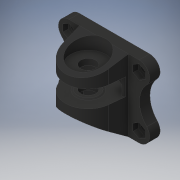
# Autodesk Inventor part: Y Bearing Mount
Saved by Autodesk Inventor 2020.2 (Build 242310000, 310)
## iProperties
Created: 2018-06-15
Part Number: Y Bearing Mount
Material: ABS Plastic
Document SubType Name: Modeling
Designer: Richard
Density: 1.06 g/cm^3
Appearance: Rubber - Black
Author: Richard
Autodesk Inventor part; units mm, degrees
ref_plane "YZ Plane" through (0, 0, 0) normal (1, 0, 0) x (0, 1, 0)
ref_plane "XZ Plane" through (0, 0, 0) normal (0, 1, 0) x (-1, 0, 0)
ref_plane "XY Plane" through (0, 0, 0) normal (0, 0, 1) x (1, 0, 0)
sketch "Sketch1" plane through (0, 0, 0) normal (0, 0, 1) x (1, 0, 0)
  line L0 (-20, -20.5) -> (20, -20.5)
  line L1 (20, -20.5) -> (20, 20.5) construction
  line L2 (20, 20.5) -> (-20, 20.5)
  line L3 (-20, 20.5) -> (-20, -20.5) construction
  line L4 (-20, -20.5) -> (20, 20.5) construction
  line L5 (20, -20.5) -> (-20, 20.5) construction
  arc A0 (-20, 20.5) -> (-24.3401, 10.3571) centre (-20, 14.5) ccw
  arc A1 (-24.3401, -10.3571) -> (-20, -20.5) centre (-20, -14.5) ccw
  arc A2 (20, -20.5) -> (24.3401, -10.3571) centre (20, -14.5) ccw
  arc A3 (24.3401, 10.3571) -> (20, 20.5) centre (20, 14.5) ccw
  arc A4 (-24.3401, -10.3571) -> (-24.3401, 10.3571) centre (-35.19, 0) ccw
  arc A5 (24.3401, 10.3571) -> (24.3401, -10.3571) centre (35.19, 0) ccw
  point P0 (0, 0)
  point P1 (-20, 14.5)
  point P2 (-20, -14.5)
  point P3 (20, 14.5)
  point P4 (20, -14.5)
  dimension "d0" = 40
  dimension "d1" = 41
  dimension "d2" = 14.5
  dimension "d3" = 14.5
  dimension "d4" = 6
  dimension "d5" = 6
  dimension "d6" = 6
  dimension "d7" = 6
  dimension "d8" = 70.38
  dimension "d9" = 35.19
  constraints: 12 end point, 12 point on circle, 8 tangent, 6 centre point, 4 point on line, 2 horizontal alignment, 2 midpoint, 2 parallel, 1 horizontal, 1 perpendicular
  measures "d0" distance of L2.end L1.end
  measures "d1" distance of L1.end L0.end
  measures "d2" vertical distance of point (0, 0) point (-20, 14.5)
  measures "d3" vertical distance of point (-20, -14.5) point (0, 0)
  measures "d4" radius of A0
  measures "d5" radius of A3
  measures "d6" radius of A2
  measures "d7" radius of A1
  measures "d8" distance of A5.centre A4.centre
  measures "d9" distance of point (0, 0) A4.centre
extrude "Extrusion1" add sketch "Sketch1" along normal blind 6
sketch "Sketch2" plane through (-20, 20.5, 0) normal (0, 1, 0) x (1, 0, 0)
  line L0 (0, -6) -> (40, -6) projected
  line L1 (6, -6) -> (7.069, -16.3372)
  arc A0 (7.069, -16.3372) -> (32.931, -16.3372) centre (20, -15) ccw
  line L2 (32.931, -16.3372) -> (34, -6)
  line L3 (40, 0) -> (0, 0) projected
  circle A1 centre (20, -15) radius 10 construction
  circle A2 centre (20, -15) radius 4.25
  point P0 (20, 0)
  point P1 (20, 0)
  dimension "d12" = 28
  dimension "d13" = 9
  dimension "d14" = 20
  dimension "d15" = 3
  dimension "d34" = 8.5
  constraints: 4 end point, 3 centre point, 2 coincident, 2 point on circle, 2 point on line, 2 tangent, 1 equal length, 1 midpoint, 1 vertical alignment
  measures "d12" distance of L2.end L1.start
  measures "d13" distance from line of L0 A0.centre
  measures "d14" diameter of A1
  measures "d15" radial gap between concentric circles of A0 A1
  measures "d34" diameter of A2
extrude "Extrusion2" add sketch "Sketch2" against normal up to surface (41 mm away)
sketch "Sketch3" plane through (0, 0, 0) normal (1, 0, 0) x (0, 1, 0)
  line L0 (-20.5, 6) -> (-20.5, 16.3372) projected
  line L1 (-20.5, 16.3372) -> (-20.5, 28) projected
  line L2 (-20.5, 16.3372) -> (-20.5, 6) projected
  line L3 (-20.5, 6) -> (-5.0954, 28)
  line L4 (20.5, 28) -> (-20.5, 28) construction
  line L5 (-5.0954, 28) -> (-20.5, 28)
  point P0 (0, 0)
  dimension "d18" = 35
  constraints: 4 end point, 1 horizontal, 1 point on line
  measures "d18" angle of L0 L3
extrude "Extrusion3" cut sketch "Sketch3" along normal mid plane 41.25
sketch "Sketch4" plane through (0, 0, 0) normal (1, 0, 0) x (0, 1, 0)
  line L0 (20.5, 16.3372) -> (20.5, 6) projected
  line L1 (20.5, 28) -> (20.5, 16.3372) projected
  line L2 (20.5, 6) -> (20.5, 16.3372) projected
  line L3 (20.5, 6) -> (14.6051, 28)
  line L4 (14.6051, 28) -> (20.5, 28)
  point P0 (0, 0)
  dimension "d21" = 15
  constraints: 4 end point, 1 perpendicular
  measures "d21" angle of L1 L3
extrude "Extrusion4" cut sketch "Sketch4" along normal mid plane 41.25
sketch "Sketch6" plane through (-20, -20.5, 0) normal (0, -1, 0) x (1, 0, 0)
  arc A0 (32.931, 16.3372) -> (7.069, 16.3372) centre (20, 15) ccw projected
  circle A1 centre (20, 15) radius 10
  point P0 (20, 0)
  dimension "d28" = 20
  constraints: 1 centre point, 1 coincident
  measures "d28" diameter of A1
extrude "Extrusion6" cut sketch "Sketch6" against normal blind 17.5
sketch "Sketch7" plane through (-20, 20.5, 0) normal (0, 1, 0) x (1, 0, 0)
  arc A0 (7.069, -16.3372) -> (32.931, -16.3372) centre (20, -15) ccw projected
  circle A1 centre (20, -15) radius 10
  point P0 (20, 0)
  dimension "d31" = 20
  constraints: 1 centre point, 1 coincident
  measures "d31" diameter of A1
extrude "Extrusion7" cut sketch "Sketch7" against normal blind 7.7
ref_plane "Work Plane1" through (-20, 9.8, 0) normal (0, 1, 0) x (1, 0, 0)
sketch "Sketch9" plane through (-20, 9.8, 0) normal (0, 1, 0) x (1, 0, 0)
  arc A0 (15.6411, -6) -> (24.3589, -6) centre (20, -15) ccw projected
  circle A1 centre (20, -15) radius 14
  point P0 (20, 0)
  dimension "d38" = 28
  constraints: 1 centre point, 1 coincident
  measures "d38" diameter of A1
extrude "Extrusion9" cut sketch "Sketch9" against normal blind 9.8
fillet "Fillet1" radius 1 2 edges at (13.4655, 4.9, 11.1686) (-13.4655, 4.9, 11.1686)
sketch "Sketch10" plane through (0, 0, 0) normal (1, 0, 0) x (0, 1, 0)
  line L0 (9.8, 19.25) -> (9.8, 10.75) projected
  line L1 (0, 10.75) -> (0, 19.25) projected
  line L2 (0, 19.25) -> (0.5, 19.25)
  line L3 (0.5, 19.25) -> (0.5, 21)
  line L4 (0.5, 21) -> (0, 22)
  line L5 (0, 22) -> (0, 19.25)
  line L6 (9.8, 19.25) -> (9.3, 19.25)
  line L7 (9.3, 19.25) -> (9.3, 21)
  line L8 (9.3, 21) -> (9.8, 22)
  line L9 (9.8, 22) -> (9.8, 19.25)
  line L10 (9.8, 15) -> (0, 15)
  point P0 (0, 0)
  dimension "d44" = 12
  dimension "d45" = 14
  dimension "d46" = 0.5
  constraints: 18 end point, 3 equal length, 2 midpoint, 2 parallel, 2 perpendicular, 2 point on line, 1 horizontal
  measures "d44" diameter of L7.end L10
  measures "d45" diameter of L8.end L10
  measures "d46" distance of L0.start L6.end
revolve "Revolution1" add sketch "Sketch10" angle 360 about axis through (0, 9.8, 15) along (0, -1, 0)
sketch "Sketch11" plane through (0, 0, 6) normal (0, 0, 1) x (1, 0, 0)
  line L0 (-14, -20.5) -> (-14, 20.5) projected
  line L1 (-14, 20.5) -> (-20, 20.5) projected
  arc A0 (-20, 20.5) -> (-24.3401, 10.3571) centre (-20, 14.5) ccw projected
  arc A1 (-24.3401, -10.3571) -> (-24.3401, 10.3571) centre (-35.19, 0) ccw projected
  arc A2 (-24.3401, -10.3571) -> (-20, -20.5) centre (-20, -14.5) ccw projected
  line L2 (-20, -20.5) -> (-14, -20.5) projected
  line L3 (14, 20.5) -> (14, -20.5) projected
  line L4 (14, -20.5) -> (20, -20.5) projected
  arc A3 (20, -20.5) -> (24.3401, -10.3571) centre (20, -14.5) ccw projected
  arc A4 (24.3401, 10.3571) -> (24.3401, -10.3571) centre (35.19, 0) ccw projected
  arc A5 (24.3401, 10.3571) -> (20, 20.5) centre (20, 14.5) ccw projected
  line L5 (20, 20.5) -> (14, 20.5) projected
  point P0 (0, 0)
hole "Hole1" at (-20, 14.5, 6) at (-20, -14.5, 6) at (20, -14.5, 6) at (20, 14.5, 6) direction (0, 0, -1) diameter 4 end through all start extended yes
sketch "Sketch12" plane through (0, 0, 6) normal (0, 0, 1) x (1, 0, 0)
  circle A0 centre (-20, 14.5) radius 2 projected
  circle A1 centre (-20, -14.5) radius 2 projected
  circle A2 centre (20, -14.5) radius 2 projected
  circle A3 centre (20, 14.5) radius 2 projected
  line L0 (-16.5, 16.5207) -> (-16.5, 12.4793)
  line L1 (-16.5, 12.4793) -> (-20, 10.4585)
  line L2 (-20, 10.4585) -> (-23.5, 12.4793)
  line L3 (-23.5, 12.4793) -> (-23.5, 16.5207)
  line L4 (-23.5, 16.5207) -> (-20, 18.5415)
  line L5 (-20, 18.5415) -> (-16.5, 16.5207)
  line L6 (23.5, 16.5207) -> (23.5, 12.4793)
  line L7 (23.5, 12.4793) -> (20, 10.4585)
  line L8 (20, 10.4585) -> (16.5, 12.4793)
  line L9 (16.5, 12.4793) -> (16.5, 16.5207)
  line L10 (16.5, 16.5207) -> (20, 18.5415)
  line L11 (20, 18.5415) -> (23.5, 16.5207)
  line L12 (23.5, -12.4793) -> (23.5, -16.5207)
  line L13 (23.5, -16.5207) -> (20, -18.5415)
  line L14 (20, -18.5415) -> (16.5, -16.5207)
  line L15 (16.5, -16.5207) -> (16.5, -12.4793)
  line L16 (16.5, -12.4793) -> (20, -10.4585)
  line L17 (20, -10.4585) -> (23.5, -12.4793)
  line L18 (-16.5, -12.4793) -> (-16.5, -16.5207)
  line L19 (-16.5, -16.5207) -> (-20, -18.5415)
  line L20 (-20, -18.5415) -> (-23.5, -16.5207)
  line L21 (-23.5, -16.5207) -> (-23.5, -12.4793)
  line L22 (-23.5, -12.4793) -> (-20, -10.4585)
  line L23 (-20, -10.4585) -> (-16.5, -12.4793)
  point P0 (0, 0)
  dimension "d55" = 7
  constraints: 48 end point, 4 coincident, 4 vertical, 3 parallel, 52 other
  measures "d55" distance between parallel lines of L19 L22
extrude "Extrusion10" cut sketch "Sketch12" against normal blind 3
sketch "Sketch13" plane through (0, -3, 15) normal (0, -1, 0) x (1, 0, 0)
  circle A0 centre (0, 0) radius 6 projected
  circle A1 centre (0, 0) radius 4.25 projected
  circle A2 centre (0, 0) radius 10 projected
  line L0 (6.75, 3.8971) -> (6.75, -3.8971)
  line L1 (6.75, -3.8971) -> (0, -7.7942)
  line L2 (0, -7.7942) -> (-6.75, -3.8971)
  line L3 (-6.75, -3.8971) -> (-6.75, 3.8971)
  line L4 (-6.75, 3.8971) -> (0, 7.7942)
  line L5 (0, 7.7942) -> (6.75, 3.8971)
  point P0 (0, -15)
  dimension "d58" = 13.5
  constraints: 12 end point, 1 coincident, 1 vertical, 13 other
  measures "d58" distance between parallel lines of L0 L3
extrude "Extrusion11" add sketch "Sketch13" along normal up to surface contours A2 surface through (0, -20.5, 6) normal (0, 0.819152, -0.5735764)
equation "\"d3\" = d2"
equation "\"d5\" = d4"
equation "\"d6\" = d5"
equation "\"d7\" = d4"
equation "\"d9\" = 0.5 * d8"
body "Solid1"
